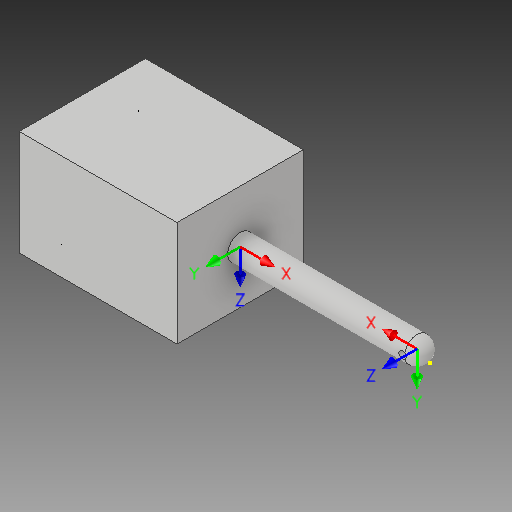
# Autodesk Inventor part: Piston Model
Saved by Autodesk Inventor 2019 (Build 230136000, 136)
## iProperties
Created: 2019-10-12
Part Number: Piston Model
Material: Generic
Document SubType Name: Modeling
Designer: sudhanva
Density: 1 g/cm^3
Appearance: Default
Author: sudhanva
Autodesk Inventor part; units mm, degrees
ref_plane "YZ Plane" through (0, 0, 0) normal (1, 0, 0) x (0, 1, 0)
ref_plane "XZ Plane" through (0, 0, 0) normal (0, 1, 0) x (-1, 0, 0)
ref_plane "XY Plane" through (0, 0, 0) normal (0, 0, 1) x (1, 0, 0)
sketch "Sketch1" plane through (0, 0, 0) normal (0, 0, 1) x (1, 0, 0)
  line L0 (-89.3385, 5.6478) -> (90.6615, 5.6478)
  line L1 (90.6615, 5.6478) -> (90.6615, -6.3522)
  line L2 (90.6615, -6.3522) -> (-89.3385, -6.3522)
  line L3 (-89.3385, -6.3522) -> (-89.3385, 5.6478)
  point P0 (0, 0)
  dimension "d0" = 180
  dimension "d1" = 12
  constraints: 8 end point, 2 parallel, 1 horizontal, 1 perpendicular
  measures "d0" distance of L1.end L2.end
  measures "d1" distance of L1.end L0.end
revolve "Revolution1" add sketch "Sketch1" angle 360 about axis through (-89.3385, 5.6478, 0) along (1, 0, 0)
sketch "Sketch2" plane through (90.6615, 5.6478, 0) normal (1, 0, 0) x (0, 0, -1)
  point P0 (0, -5.6478)
fillet "Fillet1" radius 12 1 edges at (90.6615, 17.6478, 0)
sketch "Sketch3" plane through (-89.3385, 5.6478, 0) normal (-1, 0, 0) x (0, 0, 1)
  point P0 (0, -5.6478)
sketch "Sketch4" plane through (78.6615, 5.6478, 0) normal (0, 0, 1) x (-1, 0, 0)
  circle A0 centre (1.8559, 0) radius 3.5
  point P0 (0, 0)
  dimension "d10" = 7
  constraints: 1 centre point
  measures "d10" diameter of A0
extrude "Extrusion1" cut sketch "Sketch4" along normal mid plane 80
sketch "Sketch5" plane through (-89.3385, 5.6478, 0) normal (0, -1, 0) x (1, 0, 0)
  line L0 (-0.103, -60) -> (-150.103, -60)
  line L1 (-150.103, -60) -> (-150.103, 60)
  line L2 (-150.103, 60) -> (-0.103, 60)
  line L3 (-0.103, 60) -> (-0.103, -60)
  point P0 (0, 0)
  dimension "d19" = 120
  dimension "d20" = 150
  dimension "d21" = 60
  constraints: 8 end point, 2 parallel, 1 horizontal, 1 perpendicular
  measures "d19" distance of L2.end L0.start
  measures "d20" distance of L1.end L2.end
  measures "d21" distance from line of L0 point (0, 0)
extrude "Extrusion2" add sketch "Sketch5" along normal mid plane 100
body "Solid1"
